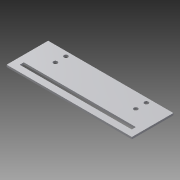
# Autodesk Inventor part: Fork 2 ver2c
Saved by Autodesk Inventor 2015 (Build 190159000, 159)
## iProperties
Created: 2015-06-22
Part Number: Fork 2 ver2c
Material: アルミニウム 5052 H32
Document SubType Name: シート メタル
Designer: kenta
Density: 2.68 g/cm^3
Sheet Metal Rule: Default_mm
Appearance: サテン
Mass: 11.4221 g
Surface Area: 63.8935 cm^2
Volume: 4.26196 cm^3
Author: kenta
Autodesk Inventor part; units mm, degrees
ref_plane "YZ Plane" through (0, 0, 0) normal (1, 0, 0) x (0, 1, 0)
ref_plane "XZ Plane" through (0, 0, 0) normal (0, 1, 0) x (-1, 0, 0)
ref_plane "XY Plane" through (0, 0, 0) normal (0, 0, 1) x (1, 0, 0)
sketch "スケッチ1" plane through (0, 0, 0) normal (0, 0, 1) x (1, 0, 0)
  line L0 (-47.5, 5.75) -> (47.5, 5.75)
  line L1 (47.5, 5.75) -> (47.5, -5.75)
  line L2 (47.5, -5.75) -> (-47.5, -5.75)
  line L3 (-47.5, -5.75) -> (-47.5, 5.75)
  line L4 (-47.5, 5.75) -> (47.5, -5.75) construction
  line L5 (47.5, 5.75) -> (-47.5, -5.75) construction
  point P0 (0, 0)
  dimension "d0" = 11.5
  dimension "d1" = 95
  constraints: 12 end point, 2 midpoint, 2 parallel, 1 horizontal, 1 perpendicular
  measures "d0" distance of L0.end L1.end
  measures "d1" distance of L1.end L2.end
extrude "押し出し1" add sketch "スケッチ1" along normal blind 1.5
sketch "スケッチ2" plane through (0, 0, 1.5) normal (0, 0, 1) x (1, 0, 0)
  line L0 (-42.5, 2.3) -> (42.5, 2.3)
  line L1 (42.5, 2.3) -> (42.5, -0.8)
  line L2 (42.5, -0.8) -> (-42.5, -0.8)
  line L3 (-42.5, -0.8) -> (-42.5, 2.3)
  line L4 (-47.5, -5.75) -> (47.5, -5.75) projected
  line L5 (47.5, -5.75) -> (47.5, 5.75) projected
  point P0 (0, 0)
  dimension "d8" = 3.1
  dimension "d9" = 85
  dimension "d10" = 4.95
  dimension "d11" = 5
  constraints: 8 end point, 2 parallel, 1 horizontal, 1 perpendicular
  measures "d8" distance of L0.end L1.end
  measures "d9" distance of L1.end L2.end
  measures "d10" distance between parallel lines of L4 L2
  measures "d11" distance between parallel lines of L1 L5
extrude "押し出し2" cut sketch "スケッチ2" against normal blind 1.5
sketch "スケッチ5" plane through (-47.5, 5.75, 0) normal (0, 1, 0) x (1, 0, 0)
  line L0 (0, 0) -> (95, 0)
  line L1 (95, 0) -> (95, -1.5)
  line L2 (95, -1.5) -> (0, -1.5)
  line L3 (0, -1.5) -> (0, 0)
  point P0 (47.5, 0)
  constraints: 8 end point, 2 parallel, 1 horizontal, 1 perpendicular
extrude "押し出し4" add sketch "スケッチ5" along normal blind 20
sketch "スケッチ6" plane through (0, 0, 1.5) normal (0, 0, 1) x (1, 0, 0)
  line L0 (-47.5, 25.75) -> (47.5, 25.75) projected
  line L1 (-47.5, -5.75) -> (-47.5, 25.75) projected
  point P0 (0, 0)
  point P1 (30.5, 22.25)
  point P2 (-30.5, 22.25)
  point P3 (-30.5, 14.25)
  point P4 (30.5, 14.25)
  dimension "d32" = 3.5
  dimension "d33" = 8
  dimension "d34" = 61
  dimension "d35" = 17
  constraints: 2 horizontal alignment, 2 vertical alignment
  measures "d32" distance from line of point (-30.5, 22.25) L0
  measures "d33" distance of point (-30.5, 22.25) point (-30.5, 14.25)
  measures "d34" distance of point (-30.5, 14.25) point (30.5, 14.25)
  measures "d35" distance from line of point (-30.5, 14.25) L1
hole "穴2" at (30.5, 22.25, 1.5) at (-30.5, 22.25, 1.5) at (-30.5, 14.25, 1.5) at (30.5, 14.25, 1.5) direction (0, 0, -1) diameter 3.1 end through all
equation "\"d41\" = Thickness"
equation "\"BendRadius\" = Thickness"
equation "\"BendReliefWidth\" = Thickness"
equation "\"BendReliefDepth\" = 0.5 * Thickness"
equation "\"CornerReliefSize\" = 4 * Thickness"
equation "\"MinimumRemnant\" = 2 * Thickness"
equation "\"TransitionRadius\" = BendRadius"
equation "\"JacobiRadiusSize\" = BendRadius"
equation "\"GapSize\" = Thickness"
equation "\"Thickness\" = 0.5"
